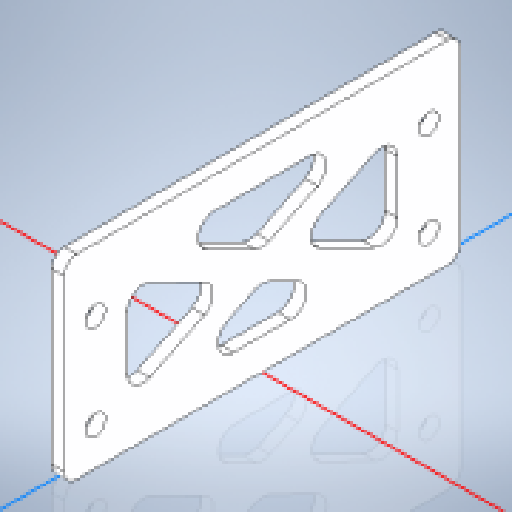
# Autodesk Inventor part: 2mm_double_for_pulley
Saved by Autodesk Inventor 2025 (Build 290162000, 162)
## iProperties
Created: 2025-02-24
Part Number: 2mm_double_for_pulley
Material: アルミニウム 6061
Document SubType Name: Modeling
Designer: Zhopa
Density: 2.7 g/cm^3
Appearance: アルミニウム - フラット
Author: Zhopa
Autodesk Inventor part; units mm, degrees
ref_plane "YZ Plane" through (0, 0, 0) normal (1, 0, 0) x (0, 1, 0)
ref_plane "XZ Plane" through (0, 0, 0) normal (0, 1, 0) x (-1, 0, 0)
ref_plane "XY Plane" through (0, 0, 0) normal (0, 0, 1) x (1, 0, 0)
sketch "Sketch1" plane through (0, 0, 0) normal (1, 0, 0) x (0, 1, 0)
  line L0 (-15.5, 31.5) -> (15.5, 31.5)
  line L1 (15.5, 31.5) -> (15.5, -31.5)
  line L2 (15.5, -31.5) -> (-15.5, -31.5)
  line L3 (-15.5, -31.5) -> (-15.5, 31.5)
  line L4 (-15.5, 31.5) -> (15.5, -31.5) construction
  line L5 (15.5, 31.5) -> (-15.5, -31.5) construction
  circle A0 centre (5.5, 26.5) radius 1.6
  circle A1 centre (5.5, -26.5) radius 1.6
  circle A2 centre (-9.5, -26.5) radius 1.6
  circle A3 centre (-9.5, 26.5) radius 1.6
  circle A4 centre (0, 10.5) radius 6
  circle A5 centre (0, -10.5) radius 6
  point P0 (0, 0)
  point P1 (-9.5, 26.5)
  point P2 (5.5, -26.5)
  point P3 (-9.5, -16)
  dimension "d0" = 63
  dimension "d1" = 31
  dimension "d2" = 5
  dimension "d3" = 10
  dimension "d5" = 15
  dimension "d6" = 5
  dimension "d7" = 3.2
  dimension "d8" = 3.2
  dimension "d9" = 3.2
  dimension "d10" = 3.2
  dimension "d15" = 5
  dimension "d16" = 5
  dimension "d17" = 5
  dimension "d18" = 21
  dimension "d19" = 21
  dimension "d20" = 12
  dimension "d21" = 12
  constraints: 12 end point, 6 centre point, 3 coincident, 2 midpoint, 2 parallel, 1 horizontal, 1 perpendicular
  measures "d0" distance of L0.end L1.end
  measures "d1" distance of L1.end L2.end
  measures "d2" distance from line of L0 point (5.5, 26.5)
  measures "d3" distance from line of point (5.5, 26.5) L1
  measures "d5" distance of point (5.5, 26.5) point (-9.5, 26.5)
  measures "d6" distance from line of L2 point (5.5, -26.5)
  measures "d7" diameter of A0
  measures "d8" diameter of A1
  measures "d9" diameter of A2
  measures "d10" diameter of A3
  measures "d15" distance from line of L0 A3.centre
  measures "d16" distance from line of L2 A1.centre
  measures "d17" distance from line of L2 A2.centre
  measures "d18" distance from line of L0 point (0, 10.5)
  measures "d19" distance from line of L2 point (0, -10.5)
  measures "d20" diameter of A4
  measures "d21" diameter of A5
extrude "Extrusion1" add sketch "Sketch1" along normal blind 2 contours L0 L1 L2 L3 | A4 | A5
fillet "Fillet1" radius 2 4 edges at (1, 15.5, 31.5) (1, -15.5, 31.5) (1, -15.5, -31.5) (1, 15.5, -31.5)
sketch "Sketch2" plane through (2, 0, 0) normal (1, 0, 0) x (0, 0, -1)
  line L0 (21.5, -10.5) -> (-21.5, -10.5)
  line L1 (-21.5, -10.5) -> (-21.5, 10.5)
  line L2 (-21.5, 10.5) -> (21.5, 10.5)
  line L3 (21.5, 10.5) -> (21.5, -10.5)
  line L4 (21.5, -10.5) -> (-21.5, 10.5) construction
  line L5 (-21.5, -10.5) -> (21.5, 10.5) construction
  line L6 (29.5, 15.5) -> (-29.5, 15.5) projected
  line L7 (-29.5, -15.5) -> (29.5, -15.5) projected
  line L8 (31.5, -13.5) -> (31.5, 13.5) projected
  line L9 (-31.5, 13.5) -> (-31.5, -13.5) projected
  line L10 (-21.5, 10.5) -> (21.5, -10.5)
  line L11 (21.5, 10.5) -> (-21.5, -10.5)
  line L12 (-21.5, 7.5) -> (15.3571, -10.5)
  line L13 (-18.5, 10.5) -> (21.5, -9.0349)
  line L14 (0, 10.5) -> (0, 6.4862)
  line L15 (21.5, 7.5) -> (-15.3571, -10.5)
  line L16 (18.5, 10.5) -> (-21.5, -9.0349)
  point P0 (0, 0)
  point P1 (0, -3)
  point P2 (-15.3571, -10.5)
  point P3 (21.5, 7.5)
  point P4 (4.5714, -0.7674)
  point P5 (0, 1.4651)
  point P6 (18.5, 10.5)
  point P7 (-21.5, -9.0349)
  point P8 (-4.5714, -0.7674)
  dimension "d22" = 5
  dimension "d23" = 5
  dimension "d24" = 10
  dimension "d25" = 10
  dimension "d26" = 3
  dimension "d27" = 3
  dimension "d31" = 180
  constraints: 26 end point, 4 point on line, 4 symmetric about line, 3 midpoint, 3 parallel, 1 collinear, 1 horizontal, 1 perpendicular, 1 vertical
  measures "d22" distance between parallel lines of L2 L6
  measures "d23" distance between parallel lines of L7 L0
  measures "d24" distance between parallel lines of L8 L3
  measures "d25" distance between parallel lines of L9 L1
  measures "d26" distance of L1.end L13.start
  measures "d27" distance of L12.start L1.end
  measures "d31" angle of L4 L12
extrude "Extrusion2" cut sketch "Sketch2" against normal blind 2 contours L0 L15 L12 | L13 L15 L3 | L1 L12 L16 | L16 L13 L2
fillet "Fillet2" radius 2.5 12 edges at (1, 7.5, 21.5) (1, 10.5, 18.5) (1, 10.5, -18.5) (1, 7.5, -21.5) (1, -9.0349, -21.5) (1, -10.5, -15.3571) (1, -3, 0) (1, 1.4651, 0) (1, -0.7674, -4.5714) (1, -0.7674, 4.5714) (1, -10.5, 15.3571) (1, -9.0349, 21.5)
equation "\"d15\" = d2"
equation "\"d16\" = d6"
equation "\"d17\" = d6"
body "Solid1"
